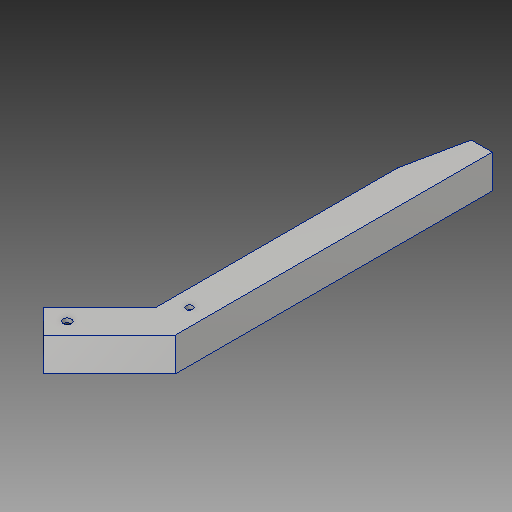
# Autodesk Inventor part: Part2
Saved by Autodesk Inventor 2017 (Build 210142000, 142)
## iProperties
Created: 2018-01-31
Part Number: Part2
Material: Aluminum 6061
Document SubType Name: Modeling
Designer: S338674153
Density: 2.7 g/cm^3
Appearance: Aluminum - Flat
Author: S338674153
Autodesk Inventor part; units mm, degrees
ref_plane "YZ Plane" through (0, 0, 0) normal (1, 0, 0) x (0, 1, 0)
ref_plane "XZ Plane" through (0, 0, 0) normal (0, 1, 0) x (-1, 0, 0)
ref_plane "XY Plane" through (0, 0, 0) normal (0, 0, 1) x (1, 0, 0)
sketch "Sketch1" plane through (0, 0, 0) normal (0, 1, 0) x (-1, 0, 0)
  line L0 (0, 0) -> (0, -228.6)
  line L1 (0, -228.6) -> (-25.4, -228.6)
  line L2 (-25.4, -228.6) -> (-25.4, 10.5159)
  line L3 (-25.4, 10.5159) -> (24.2621, 60.178)
  line L4 (24.2621, 60.178) -> (42.5226, 42.5226)
  line L5 (42.5226, 42.5226) -> (0, 0)
  dimension "d0" = 228.6
  dimension "d1" = 25.4
  dimension "d2" = 135
  dimension "d3" = 25.4
  constraints: 12 end point, 2 perpendicular, 1 parallel, 1 vertical
  measures "d0" distance of L0.start L0.end
  measures "d1" distance of L0.end L1.end
  measures "d2" angle of L3 L2
  measures "d3" distance of L3.end L4.end
extrude "Extrusion1" add sketch "Sketch1" along normal blind 25.4
sketch "Sketch2" plane through (0, 25.4, 0) normal (0, 1, 0) x (1, 0, 0)
  line L0 (25.4, 228.6) -> (0, 228.6) projected
  line L1 (9.525, 228.6) -> (0, 182.5245)
  line L2 (0, 228.6) -> (0, 0) projected
  dimension "d6" = 11.68
  dimension "d7" = 9.525
  constraints: 2 end point, 2 point on line
  measures "d6" angle of L1 L2
  measures "d7" distance of L1.start L0.end
extrude "Extrusion2" cut sketch "Sketch2" against normal through all
shell "Shell1" thickness 3.175 removed faces 3 at (3.175, 16.9333, -197.883) at (14.8167, 8.4667, -228.6) at (-30.3489, 8.4667, 54.2929)
sketch "Sketch3" plane through (0, 25.4, 0) normal (0, 1, 0) x (1, 0, 0)
  circle A0 centre (-24.4095, -42.3701) radius 3.175
  line L0 (-42.5226, -42.5226) -> (-24.2621, -60.178) projected
  line L1 (0, 0) -> (-42.5226, -42.5226) projected
  line L2 (0, 0) -> (25.4, 0)
  line L3 (25.4, -10.5159) -> (25.4, 228.6) projected
  circle A1 centre (12.7, 12.7) radius 2.54
  line L4 (0, 182.5245) -> (0, 0) projected
  dimension "d11" = 6.35
  dimension "d12" = 12.7
  dimension "d13" = 12.7
  dimension "d14" = 5.08
  dimension "d15" = 12.7
  dimension "d16" = 12.7
  constraints: 2 centre point, 2 end point, 1 horizontal, 1 point on line
  measures "d11" diameter of A0
  measures "d12" distance from line of A0.centre L0
  measures "d13" distance from line of A0.centre L1
  measures "d14" diameter of A1
  measures "d15" distance from line of A1.centre L2
  measures "d16" distance from line of L4 A1.centre
extrude "Extrusion3" cut sketch "Sketch3" against normal through all
body "Solid1"
